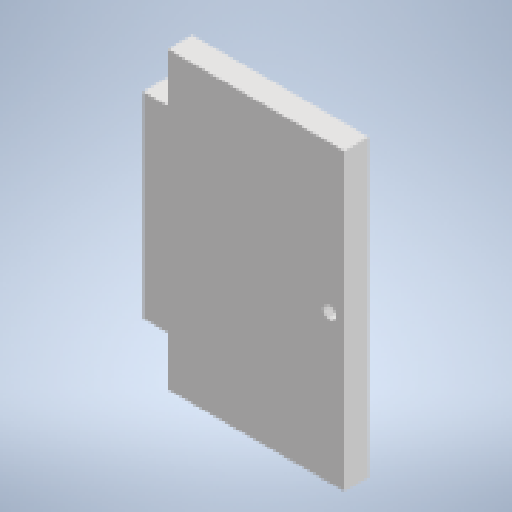
# Autodesk Inventor part: pin holder
Saved by Autodesk Inventor 2023 (Build 270158000, 158)
## iProperties
Created: 2023-10-15
Part Number: pin holder
Material: Generic
Document SubType Name: Modeling
Designer: Nate
Density: 1 g/cm^3
Appearance: Default
Author: Nate
Autodesk Inventor part; units mm, degrees
ref_plane "YZ Plane" through (0, 0, 0) normal (1, 0, 0) x (0, 1, 0)
ref_plane "XZ Plane" through (0, 0, 0) normal (0, 1, 0) x (-1, 0, 0)
ref_plane "XY Plane" through (0, 0, 0) normal (0, 0, 1) x (1, 0, 0)
sketch "Sketch1" plane through (0, 0, 0) normal (0, 0, 1) x (1, 0, 0)
  line L0 (0, 0) -> (6.35, 0)
  line L1 (6.35, 0) -> (6.35, -50.8)
  line L2 (6.35, -50.8) -> (0, -50.8)
  line L3 (0, -50.8) -> (0, 0)
  line L4 (52.07, 12.7) -> (6.35, 12.7)
  line L5 (6.35, 12.7) -> (6.35, -63.5)
  line L6 (6.35, -63.5) -> (52.07, -63.5)
  line L7 (52.07, -63.5) -> (52.07, 12.7)
  circle A0 centre (48.2346, -25.4) radius 1.5875
  dimension "d0" = 6.35
  dimension "d1" = 50.8
  dimension "d2" = 76.2
  dimension "d3" = 12.7
  dimension "d4" = 45.72
  dimension "d5" = 3.175
  dimension "d6" = 38.1
  dimension "d7" = 41.8846
  constraints: 16 end point, 4 parallel, 2 horizontal, 2 perpendicular, 1 centre point
  measures "d0" distance of L1.end L2.end
  measures "d1" distance of L0.end L1.end
  measures "d2" distance of L4.end L5.end
  measures "d3" distance between parallel lines of L6 L2
  measures "d4" distance between parallel lines of L7 L5
  measures "d5" diameter of A0
  measures "d6" distance from line of A0.centre L4
  measures "d7" distance from line of L1 A0.centre
extrude "Extrusion1" add sketch "Sketch1" along normal blind 6.35
body "Solid1"
